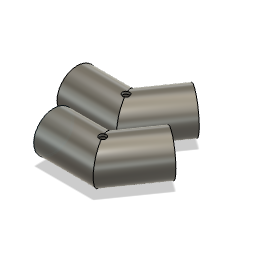
bottom connector 125 v3 (Autodesk Fusion 360 design; units mm, degrees)
Autodesk Fusion 360 part; units mm, degrees
sketch "Sketch1" plane through (0, 0, 0) normal (0, 1, 0) x (1, 0, 0)
  line L0 (0, 0) -> (50, 0)
  line L1 (50, 0) -> (78.6788, 40.9576)
  dimension "d1" = 125
  dimension "d2" = 50
  constraint coincident L0.start origin
  constraint horizontal L0
  measures "d1" angle of L0 L1
  measures "d2" distance of L0.end L1.end
pipe "Pipe1" add diameter 41 wall 2 path "Sketch1" along L0 L1 in component "Component"
sketch "Sketch2" plane through (0, 0, 0) normal (-1, 0, 0) x (0, 0, 1)
  circle A0 centre (0, 0) radius 18.5
  circle A1 centre (0, 0) radius 20.5
sketch "Sketch3" plane through (0, 0, 0) normal (0, 1, 0) x (1, 0, 0)
  circle A0 centre (50, 0) radius 3.5
  dimension "d7" = 7
  measures "d7" diameter of A0
extrude "Extrude1" cut sketch "Sketch3" along normal blind 35 and the other way blind 45 in component "Component"
sketch "Sketch4" plane through (0, 0, 0) normal (0, 1, 0) x (1, 0, 0)
  line L0 (50, 0) -> (-5, 0)
  line L1 (50, 0) -> (78.7509, 41.0606)
  line L2 (50, 0) -> (100.1257, 0) construction
  dimension "d12" = 55
  constraint horizontal L0
  constraint horizontal L2
  measures "d12" angle of L1 L2
pipe "Pipe2" add diameter 38 wall 1 path "Sketch4" along L1 L0 in component "Component"
delete_face "DeleteFace1" 1 faces at (-1.6667, 18.9056, -1.8918) in component "Component"
sketch "Sketch5" plane through (0, 0, 0) normal (0, 1, 0) x (1, 0, 0)
  circle A0 centre (50, 0) radius 3.5
  dimension "d17" = 7
  measures "d17" diameter of A0
extrude "Extrude2" cut sketch "Sketch5" along normal blind 105 and the other way blind 35 in component "Component"
component "Component" placed x (1, 0, 0) y (0, 1, 0) z (0, 0, 1) at (0, 0, 0)
component "Component" placed x (1, 0, 0) y (0, 1, 0) z (0, 0, 1) at (-25.6148, 0, -49.4321)
